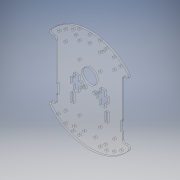
# Autodesk Inventor part: TopPlate
Saved by Autodesk Inventor 2018 (Build 220112000, 112)
## iProperties
Created: 2018-01-11
Part Number: TopPlate
Material: Polycarbonate, Clear
Document SubType Name: Modeling
Designer: Kyle
Density: 1.2 g/cm^3
Appearance: Polycarbonate - Clear
Author: Kyle
Autodesk Inventor part; units mm, degrees
ref_plane "YZ Plane" through (0, 0, 0) normal (1, 0, 0) x (0, 1, 0)
ref_plane "XZ Plane" through (0, 0, 0) normal (0, 1, 0) x (-1, 0, 0)
ref_plane "XY Plane" through (0, 0, 0) normal (0, 0, 1) x (1, 0, 0)
sketch "Sketch1" plane through (0, 0, 0) normal (0, 0, 1) x (1, 0, 0)
  circle A0 centre (0, 0) radius 69.85
  dimension "d0" = 139.7
  constraints: 1 centre point, 1 coincident
  measures "d0" diameter of A0
extrude "Extrusion1" add sketch "Sketch1" along normal blind 2.54
sketch "Sketch2" plane through (0, 0, 2.54) normal (0, 0, 1) x (1, 0, 0)
  circle A0 centre (0, 0) radius 69.85 projected
  circle A1 centre (0, 16.51) radius 10.16
  point P0 (0, 69.85)
  dimension "d97" = 53.34
  dimension "d98" = 20.32
  constraints: 1 centre point, 1 vertical alignment, 2 other
  measures "d97" distance of A1.centre point (0, 69.85)
  measures "d98" diameter of A1
sketch "Sketch3" plane through (0, 0, 2.54) normal (0, 0, 1) x (1, 0, 0)
  circle A0 centre (0, 0) radius 69.85 projected
  circle A1 centre (33.655, 40.9575) radius 1.5875
  circle A2 centre (-33.02, 40.9575) radius 1.5875
  circle A3 centre (33.655, -40.9575) radius 1.5875
  circle A4 centre (-33.02, -40.9575) radius 1.5875
  point P0 (0, 69.85)
  point P1 (69.85, 0)
  point P2 (0, -69.85)
  point P3 (-69.85, 0)
  dimension "d22" = 3.175
  dimension "d28" = 3.175
  constraints: 4 centre point, 4 point on circle, 4 other
  measures "d22" diameter of A1
  measures "d28" diameter of A2
extrude "Extrusion4" cut sketch "Sketch3" against normal blind 25.4 contours A1 | A2 | A3 | A4
extrude "Extrusion5" cut sketch "Sketch2" against normal blind 25.4 contours A1
sketch "Sketch4" plane through (0, 0, 2.54) normal (0, 0, 1) x (1, 0, 0)
  circle A0 centre (0, 65.7225) radius 1.5875
  circle A1 centre (0, 0) radius 69.85 projected
  circle A2 centre (13.97, 65.7225) radius 1.5875
  circle A3 centre (-13.97, 65.7225) radius 1.5875
  circle A4 centre (0, 55.5625) radius 1.5875
  circle A5 centre (19.05, 55.5625) radius 1.5875
  circle A6 centre (-19.05, 55.5625) radius 1.5875
  circle A7 centre (33.02, 55.5625) radius 1.5875
  circle A8 centre (-33.02, 55.5625) radius 1.5875
  circle A9 centre (22.86, 60.6425) radius 1.5875
  circle A10 centre (-22.86, 60.6425) radius 1.5875
  circle A11 centre (41.91, 49.2125) radius 1.5875
  circle A12 centre (-41.91, 49.2125) radius 1.5875
  circle A13 centre (13.97, 51.7525) radius 1.5875
  circle A14 centre (-13.97, 51.7525) radius 1.5875
  circle A15 centre (-13.97, 28.8925) radius 1.5875
  circle A16 centre (13.97, 28.8925) radius 1.5875
  line L0 (6.0325, 1.5875) -> (7.9375, 1.5875)
  line L1 (9.525, 0) -> (9.525, 0)
  line L2 (7.9375, -1.5875) -> (6.0325, -1.5875)
  line L3 (4.445, 0) -> (4.445, 0)
  line L4 (-7.9375, 1.5875) -> (-6.0325, 1.5875)
  line L5 (-4.445, 0) -> (-4.445, 0)
  line L6 (-6.0325, -1.5875) -> (-7.9375, -1.5875)
  line L7 (-9.525, 0) -> (-9.525, 0)
  line L8 (25.4, 3.81) -> (25.4, -3.81)
  line L9 (10.795, -3.81) -> (10.795, 3.81)
  line L10 (14.605, 10.16) -> (21.59, 10.16)
  line L11 (21.59, -10.16) -> (14.605, -10.16)
  line L12 (10.795, 3.81) -> (14.605, 3.81)
  line L13 (21.59, 3.81) -> (25.4, 3.81)
  line L14 (14.605, -10.16) -> (14.605, -3.81)
  line L15 (14.605, 3.81) -> (14.605, 10.16)
  line L16 (21.59, 10.16) -> (21.59, 3.81)
  line L17 (21.59, -3.81) -> (21.59, -10.16)
  line L18 (25.4, -3.81) -> (21.59, -3.81)
  line L19 (14.605, -3.81) -> (10.795, -3.81)
  line L20 (-10.795, 3.81) -> (-10.795, -3.81)
  line L21 (-25.4, -3.81) -> (-25.4, 3.81)
  line L22 (-21.59, 10.16) -> (-14.605, 10.16)
  line L23 (-14.605, -10.16) -> (-21.59, -10.16)
  line L24 (-25.4, 3.81) -> (-21.59, 3.81)
  line L25 (-14.605, 3.81) -> (-10.795, 3.81)
  line L26 (-21.59, -10.16) -> (-21.59, -3.81)
  line L27 (-21.59, 3.81) -> (-21.59, 10.16)
  line L28 (-14.605, 10.16) -> (-14.605, 3.81)
  line L29 (-14.605, -3.81) -> (-14.605, -10.16)
  line L30 (-10.795, -3.81) -> (-14.605, -3.81)
  line L31 (-21.59, -3.81) -> (-25.4, -3.81)
  line L32 (21.59, -13.97) -> (24.765, -13.97)
  line L33 (24.765, -13.97) -> (24.765, -26.67)
  line L34 (24.765, -26.67) -> (21.59, -26.67)
  line L35 (21.59, -26.67) -> (21.59, -13.97)
  line L36 (-21.59, -13.97) -> (-24.765, -13.97)
  line L37 (-24.765, -13.97) -> (-24.765, -26.67)
  line L38 (-24.765, -26.67) -> (-21.59, -26.67)
  line L39 (-21.59, -26.67) -> (-21.59, -13.97)
  circle A17 centre (-13.97, -37.1475) radius 1.5875
  circle A18 centre (13.97, -37.1475) radius 1.5875
  circle A19 centre (-13.97, -60.0075) radius 1.5875
  circle A20 centre (13.97, -60.0075) radius 1.5875
  circle A21 centre (22.86, -60.0075) radius 1.5875
  circle A22 centre (-22.86, -60.0075) radius 1.5875
  circle A23 centre (21.59, -53.6575) radius 1.5875
  circle A24 centre (-21.59, -53.6575) radius 1.5875
  circle A25 centre (7.62, -52.3875) radius 1.5875
  circle A26 centre (-7.62, -52.3875) radius 1.5875
  circle A27 centre (33.02, -56.1975) radius 1.5875
  circle A28 centre (-33.02, -56.1975) radius 1.5875
  circle A29 centre (43.18, -49.8475) radius 1.5875
  circle A30 centre (-43.18, -49.8475) radius 1.5875
  arc A31 (-7.9375, 1.5875) -> (-9.525, 0) centre (-7.9375, 0) ccw
  arc A32 (-9.525, 0) -> (-7.9375, -1.5875) centre (-7.9375, 0) ccw
  arc A33 (-6.0325, -1.5875) -> (-4.445, 0) centre (-6.0325, 0) ccw
  arc A34 (-4.445, 0) -> (-6.0325, 1.5875) centre (-6.0325, 0) ccw
  arc A35 (6.0325, 1.5875) -> (4.445, 0) centre (6.0325, 0) ccw
  arc A36 (9.525, 0) -> (7.9375, 1.5875) centre (7.9375, 0) ccw
  arc A37 (7.9375, -1.5875) -> (9.525, 0) centre (7.9375, 0) ccw
  arc A38 (4.445, 0) -> (6.0325, -1.5875) centre (6.0325, 0) ccw
  point P0 (0, 69.85)
  point P1 (4.445, 1.5875)
  point P2 (9.525, -1.5875)
  point P3 (9.525, 1.5875)
  point P4 (-9.525, 1.5875)
  point P5 (-4.445, 1.5875)
  point P6 (-9.525, -1.5875)
  point P7 (-10.795, 3.8227)
  point P8 (-13.97, -37.1475)
  dimension "d101" = 3.175
  dimension "d102" = 4.1275
  dimension "d103" = 3.175
  dimension "d104" = 13.97
  dimension "d105" = 3.175
  dimension "d106" = 13.97
  dimension "d107" = 3.175
  dimension "d108" = 10.16
  dimension "d109" = 19.05
  dimension "d110" = 3.175
  dimension "d111" = 19.05
  dimension "d112" = 3.175
  dimension "d113" = 33.02
  dimension "d114" = 3.175
  dimension "d115" = 33.02
  dimension "d116" = 3.175
  dimension "d117" = 8.89
  dimension "d118" = 3.175
  dimension "d119" = 5.08
  dimension "d120" = 5.08
  dimension "d121" = 8.89
  dimension "d122" = 3.175
  dimension "d123" = 8.89
  dimension "d124" = 6.35
  dimension "d125" = 3.175
  dimension "d126" = 8.89
  dimension "d127" = 6.35
  dimension "d128" = 3.175
  dimension "d129" = 3.175
  dimension "d130" = 3.175
  dimension "d131" = 13.97
  dimension "d132" = 13.97
  dimension "d133" = 3.175
  dimension "d134" = 3.175
  dimension "d135" = 22.86
  dimension "d136" = 22.86
  dimension "d137" = 5.08
  dimension "d138" = 3.175
  dimension "d139" = 5.08
  dimension "d140" = 3.175
  dimension "d141" = 4.445
  dimension "d142" = 4.445
  dimension "d143" = 1.5875
  dimension "d144" = 1.27
  dimension "d145" = 14.605
  dimension "d146" = 7.62
  dimension "d148" = 20.32
  dimension "d149" = 6.985
  dimension "d150" = 10.16
  dimension "d152" = 2.2352
  dimension "d153" = 1.27
  dimension "d154" = 14.605
  dimension "d155" = 7.62
  dimension "d156" = 20.32
  dimension "d157" = 6.985
  dimension "d158" = 12.7
  dimension "d159" = 3.175
  dimension "d160" = 3.81
  dimension "d161" = 3.175
  dimension "d162" = 66.04
  dimension "d163" = 3.175
  dimension "d164" = 3.175
  dimension "d165" = 3.175
  dimension "d166" = 3.175
  constraints: 80 end point, 38 centre point, 28 parallel, 16 point on circle, 16 tangent, 13 point on line, 12 perpendicular, 10 horizontal, 7 equal radius, 1 collinear, 1 vertical alignment, 6 other
  measures "d101" diameter of A0
  measures "d102" distance of A0.centre point (0, 69.85)
  measures "d103" diameter of A2
  measures "d104" distance of A2.centre A0.centre
  measures "d105" diameter of A3
  measures "d106" distance of A3.centre A0.centre
  measures "d107" diameter of A4
  measures "d108" distance of A0.centre A4.centre
  measures "d109" distance of A4.centre A5.centre
  measures "d110" diameter of A5
  measures "d111" distance of A6.centre A4.centre
  measures "d112" diameter of A6
  measures "d113" distance of A7.centre A4.centre
  measures "d114" diameter of A7
  measures "d115" distance of A8.centre A4.centre
  measures "d116" diameter of A8
  measures "d117" horizontal distance of A2.centre A9.centre
  measures "d118" diameter of A9
  measures "d119" vertical distance of A2.centre A9.centre
  measures "d120" vertical distance of A10.centre A3.centre
  measures "d121" horizontal distance of A10.centre A3.centre
  measures "d122" diameter of A10
  measures "d123" horizontal distance of A7.centre A11.centre
  measures "d124" vertical distance of A11.centre A7.centre
  measures "d125" diameter of A11
  measures "d126" horizontal distance of A12.centre A8.centre
  measures "d127" vertical distance of A12.centre A8.centre
  measures "d128" diameter of A12
  measures "d129" diameter of A13
  measures "d130" diameter of A14
  measures "d131" distance of A14.centre A3.centre
  measures "d132" distance of A2.centre A13.centre
  measures "d133" diameter of A16
  measures "d134" diameter of A15
  measures "d135" distance of A15.centre A14.centre
  measures "d136" distance of A13.centre A16.centre
  measures "d137" distance of point (4.445, 1.587) point (9.525, 1.587)
  measures "d138" distance of point (9.525, 1.587) point (9.525, -1.588)
  measures "d139" distance of point (-9.525, 1.587) point (-4.445, 1.587)
  measures "d140" distance of point (-9.525, -1.588) point (-9.525, 1.587)
  measures "d141" distance from line of point (0, 0) L3
  measures "d142" distance from line of L5 point (0, 0)
  measures "d143" distance from line of point (0, 0) L0
  measures "d144" distance between parallel lines of L1 L9
  measures "d145" distance of L9.end L8.start
  measures "d146" distance of L8.start L8.end
  measures "d148" distance of L10.end L11.start
  measures "d149" distance of L11.start L11.end
  measures "d150" distance from line of point (0, 0) L10
  measures "d152" distance from line of point (-10.795, 3.823) L4
  measures "d153" distance from line of point (-10.795, 3.823) L7
  measures "d154" distance of L21.end L25.end
  measures "d155" distance of L25.end L20.end
  measures "d156" distance of L22.end L23.start
  measures "d157" distance of L23.start L26.start
  measures "d158" distance of L34.end L32.start
  measures "d159" distance of L33.end L34.end
  measures "d160" distance between parallel lines of L11 L32
  measures "d161" distance of L37.end L38.end
  measures "d162" distance of point (-13.97, -37.147) A15.centre
  measures "d163" diameter of A18
  measures "d164" diameter of A17
  measures "d165" diameter of A20
  measures "d166" diameter of A19
extrude "Extrusion6" cut sketch "Sketch4" against normal blind 2.54 contours A0 | A2 | A3 | A4 | A5 | A6 | A7 | A8 | A9 | A10 | A11 | A12 | A13 | A14 | A15 | A16 | L0 A36 A37 L2 A38 A35 | L4 A34 A33 L6 A32 A31 | L8 L18 L17 L11 L14 L19 L9 L12 L15 L10 L16 L13 | L20 L30 L29 L23 L26 L31 L21 L24 L27 L22 L28 L25 | L32 L33 L34 L35 | L39 L38 L37 L36 | A17 | A18 | A19 | A20 | A21 | A22 | A23 | A24 | A25 | A26 | A27 | A28 | A29 | A30
sketch "Sketch5" plane through (0, 0, 2.54) normal (0, 0, 1) x (1, 0, 0)
  line L0 (43.18, -13.97) -> (45.085, -13.97)
  line L1 (45.085, -26.67) -> (43.18, -26.67)
  line L2 (43.18, -26.67) -> (43.18, -13.97)
  line L3 (21.59, -13.97) -> (24.765, -13.97) projected
  line L4 (24.765, -26.67) -> (21.59, -26.67) projected
  line L5 (24.765, -13.97) -> (24.765, -26.67) projected
  line L6 (45.085, -26.67) -> (45.085, -39.37)
  circle A0 centre (0, 0) radius 69.85 projected
  line L7 (57.6977, -39.37) -> (45.085, -39.37)
  line L8 (45.085, -13.97) -> (45.085, 40.005)
  line L9 (45.085, 40.005) -> (57.2593, 40.005)
  arc A1 (57.6977, -39.37) -> (57.2593, 40.005) centre (0, 0) ccw
  line L10 (0, 0) -> (0, -8.6932)
  line L11 (-43.18, -13.97) -> (-45.085, -13.97)
  line L12 (-45.085, -26.67) -> (-43.18, -26.67)
  line L13 (-43.18, -26.67) -> (-43.18, -13.97)
  line L14 (-45.085, -26.67) -> (-45.085, -39.37)
  line L15 (-57.6977, -39.37) -> (-45.085, -39.37)
  line L16 (-45.085, -13.97) -> (-45.085, 40.005)
  line L17 (-45.085, 40.005) -> (-57.2593, 40.005)
  arc A2 (-57.2593, 40.005) -> (-57.6977, -39.37) centre (0, 0) ccw
  dimension "d199" = 18.415
  dimension "d200" = 1.905
  dimension "d201" = 12.7
  dimension "d203" = 53.975
  dimension "d205" = 12.1743
  constraints: 30 end point, 8 symmetric about line, 6 point on circle, 3 vertical, 2 centre point, 2 collinear, 2 horizontal, 1 concentric, 1 parallel, 1 other
  measures "d199" distance between parallel lines of L5 L2
  measures "d200" distance of L0.start L0.end
  measures "d201" distance from line of L1 L6.end
  measures "d203" distance from line of L0 L8.end
  measures "d205" distance of L9.end L8.end
extrude "Extrusion7" cut sketch "Sketch5" against normal blind 2.54 contours L0 L8 L9 A0 L7 L6 L1 L2 | L17 L16 L11 L13 L12 L14 L15 A0
fillet "Fillet1" radius 3.175 4 edges at (45.085, -39.37, 1.27) (-45.085, -39.37, 1.27) (-45.085, 40.005, 1.27) (45.085, 40.005, 1.27)
fillet "Fillet2" radius 3.175 4 edges at (57.2593, 40.005, 1.27) (57.6977, -39.37, 1.27) (-57.6977, -39.37, 1.27) (-57.2593, 40.005, 1.27)
body "Solid1"
